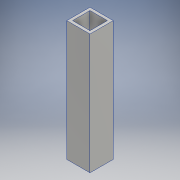
# Autodesk Inventor part: ST01
Saved by Autodesk Inventor 2017 (Build 210142000, 142)
## iProperties
Created: 2019-05-24
Part Number: ST01
Material: Aluminum 6061
Document SubType Name: Modeling
Designer: Dell
Density: 2.7 g/cm^3
Appearance: Aluminum - Flat
Mass: 801.877 g
Surface Area: 957.986 cm^2
Volume: 296.991 cm^3
Author: Dell
Autodesk Inventor part; units mm, degrees
ref_plane "YZ Plane" through (0, 0, 0) normal (1, 0, 0) x (0, 1, 0)
ref_plane "XZ Plane" through (0, 0, 0) normal (0, 1, 0) x (-1, 0, 0)
ref_plane "XY Plane" through (0, 0, 0) normal (0, 0, 1) x (1, 0, 0)
sketch "Sketch1" plane through (0, 0, 0) normal (0, 0, 1) x (1, 0, 0)
  line L0 (0, 0) -> (50.8, 0)
  line L1 (50.8, 0) -> (50.8, 50.8)
  line L2 (50.8, 50.8) -> (0, 50.8)
  line L3 (0, 50.8) -> (0, 0)
  line L4 (6.35, 6.35) -> (44.45, 6.35)
  line L5 (44.45, 6.35) -> (44.45, 44.45)
  line L6 (44.45, 44.45) -> (6.35, 44.45)
  line L7 (6.35, 44.45) -> (6.35, 6.35)
  dimension "d0" = 50.8
  dimension "d1" = 50.8
  dimension "d2" = 6.35
  constraints: 16 end point, 4 parallel, 2 perpendicular, 1 horizontal, 3 other
  measures "d0" distance of L2.end L1.end
  measures "d1" distance of L1.end L0.end
  measures "d2" distance between parallel lines of L3 L7
extrude "Extrusion1" add sketch "Sketch1" along normal blind 263.05
body "Solid1"
